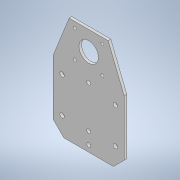
# Autodesk Inventor part: Z-Axis - Back Plate
Saved by Autodesk Inventor 2022 (Build 260153000, 153)
## iProperties
Created: 2023-01-04
Part Number: Z-Axis - Back Plate
Material: Generic
Document SubType Name: Modeling
Designer: Gaming
Density: 1 g/cm^3
Appearance: Default
Author: Gaming
Autodesk Inventor part; units mm, degrees
ref_plane "YZ Plane" through (0, 0, 0) normal (1, 0, 0) x (0, 1, 0)
ref_plane "XZ Plane" through (0, 0, 0) normal (0, 1, 0) x (-1, 0, 0)
ref_plane "XY Plane" through (0, 0, 0) normal (0, 0, 1) x (1, 0, 0)
sketch "Sketch1" plane through (0, 0, 0) normal (0, 0, 1) x (1, 0, 0)
  line L0 (-40, 60) -> (40, 60)
  line L1 (40, 60) -> (40, -60)
  line L2 (40, -60) -> (-40, -60)
  line L3 (-40, -60) -> (-40, 60)
  line L4 (-40, 60) -> (40, -60) construction
  line L5 (40, 60) -> (-40, -60) construction
  point P0 (0, 0)
  dimension "d0" = 80
  dimension "d1" = 120
  constraints: 12 end point, 2 midpoint, 2 parallel, 1 horizontal, 1 perpendicular
  measures "d0" distance of L1.end L2.end
  measures "d1" distance of L0.end L1.end
extrude "Extrusion1" add sketch "Sketch1" along normal blind 3
sketch "Sketch2" plane through (0, 0, 3) normal (0, 0, 1) x (1, 0, 0)
  line L0 (-40, -60) -> (40, -60) projected
  line L1 (-40, 60) -> (-40, -60) projected
  point P0 (0, 0)
  point P1 (-30, -39)
  point P2 (30, -39)
  point P3 (-30, 1)
  point P4 (30, 1)
  dimension "d4" = 21
  dimension "d5" = 10
  dimension "d6" = 40
  dimension "d7" = 60
  constraints: 2 horizontal alignment, 2 vertical alignment
  measures "d4" distance from line of point (-30, -39) L0
  measures "d5" distance from line of L1 point (-30, -39)
  measures "d6" distance of point (-30, 1) point (-30, -39)
  measures "d7" distance of point (30, -39) point (-30, -39)
hole "Hole1" at (-30, -39, 3) at (30, -39, 3) at (-30, 1, 3) at (30, 1, 3) direction (0, 0, -1) diameter 5.1 end through all
sketch "Sketch3" plane through (0, 0, 3) normal (0, 0, 1) x (1, 0, 0)
  circle A0 centre (0, 38) radius 11
  point P0 (0, 0)
  dimension "d15" = 22
  dimension "d16" = 38
  constraints: 1 centre point, 1 vertical alignment
  measures "d15" diameter of A0
  measures "d16" distance of A0.centre point (0, 0)
extrude "Extrusion2" cut sketch "Sketch3" against normal through all
sketch "Sketch4" plane through (0, 0, 3) normal (0, 0, 1) x (1, 0, 0)
  circle A0 centre (0, 38) radius 11 projected
  line L0 (-15.5, 53.5) -> (15.5, 53.5)
  line L1 (15.5, 53.5) -> (15.5, 22.5)
  line L2 (15.5, 22.5) -> (-15.5, 22.5)
  line L3 (-15.5, 22.5) -> (-15.5, 53.5)
  line L4 (-15.5, 53.5) -> (15.5, 22.5) construction
  line L5 (15.5, 53.5) -> (-15.5, 22.5) construction
  point P0 (0, 0)
  dimension "d19" = 31
  dimension "d20" = 31
  constraints: 12 end point, 2 midpoint, 2 parallel, 1 horizontal, 1 perpendicular
  measures "d19" distance of L1.end L2.end
  measures "d20" distance of L0.end L1.end
hole "Hole2" at (-15.5, 53.5, 3) at (-15.5, 22.5, 3) at (15.5, 22.5, 3) at (15.5, 53.5, 3) direction (0, 0, -1) diameter 3.5 end through all
sketch "Sketch5" plane through (0, 0, 3) normal (0, 0, 1) x (1, 0, 0)
  line L0 (40, 60) -> (-40, 60) projected
  line L1 (-22, 60) -> (-40, 15)
  line L2 (-40, 60) -> (-40, -60) projected
  line L3 (22, 60) -> (40, 15)
  line L4 (40, -60) -> (40, 60) projected
  point P0 (0, 0)
  dimension "d28" = 15
  dimension "d29" = 15
  dimension "d30" = 18
  dimension "d31" = 18
  dimension "d32" = 44
  constraints: 4 end point, 4 point on line
  measures "d28" vertical distance of L1.end point (0, 0)
  measures "d29" vertical distance of L3.end point (0, 0)
  measures "d30" distance from line of L1.start L2
  measures "d31" distance from line of L3.start L4
  measures "d32" distance of L3.start L1.start
extrude "Extrusion3" cut sketch "Sketch5" against normal through all
sketch "Sketch7" plane through (0, 0, 0) normal (0, 0, -1) x (-1, 0, 0)
  line L0 (40, -60) -> (-40, -60) projected
  point P0 (0, 0)
  point P1 (0, -39.5)
  dimension "d41" = 20.5
  constraints: 1 vertical alignment
  measures "d41" distance from line of point (0, -39.5) L0
hole "Hole3" at (0, -39.5, 0) direction (0, 0, 1) diameter 4.5 end through all
chamfer "Chamfer1" distance 12 angle 45 2 edges at (-40, -60, 1.5) (40, -60, 1.5)
sketch "Sketch11" plane through (0, 0, 3) normal (0, 0, 1) x (1, 0, 0)
  line L0 (-28, -60) -> (28, -60) projected
  circle A0 centre (0, 38) radius 11 projected
  point P0 (0, 0)
  point P1 (0, 8)
  point P2 (0, -53)
  dimension "d67" = 7
  dimension "d68" = 30
  constraints: 2 vertical alignment
  measures "d67" distance from line of point (0, -53) L0
  measures "d68" distance of A0.centre point (0, 8)
hole "Hole5" at (0, 8, 3) at (0, -53, 3) direction (0, 0, -1) diameter 4.5 end through all
equation "\"d29\" = d28"
equation "\"d31\" = d30"
body "Solid1"
